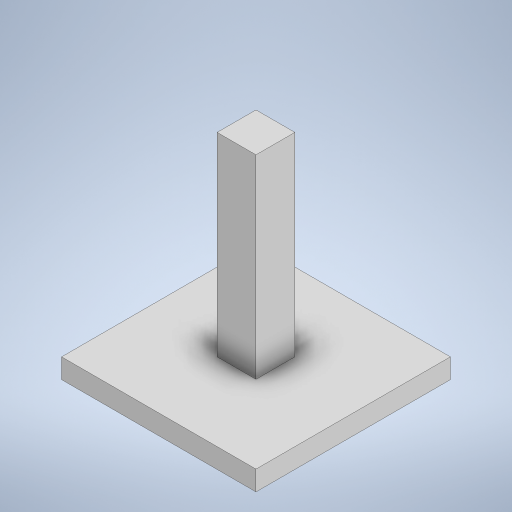
# Autodesk Inventor part: Post
Saved by Autodesk Inventor 2024 (Build 280153000, 153)
## iProperties
Created: 2024-01-14
Part Number: Post
Material: Generic
Document SubType Name: Modeling
Designer: Owner
Density: 1 g/cm^3
Appearance: Default
Author: Owner
Autodesk Inventor part; units mm, degrees
ref_plane "YZ Plane" through (0, 0, 0) normal (1, 0, 0) x (0, 1, 0)
ref_plane "XZ Plane" through (0, 0, 0) normal (0, 1, 0) x (-1, 0, 0)
ref_plane "XY Plane" through (0, 0, 0) normal (0, 0, 1) x (1, 0, 0)
sketch "Sketch1" plane through (0, 0, 0) normal (0, 1, 0) x (-1, 0, 0)
  line L0 (0, 0) -> (500, 0)
  line L1 (500, 0) -> (500, -500)
  line L2 (500, -500) -> (0, -500)
  line L3 (0, -500) -> (0, 0)
  dimension "d0" = 500
  dimension "d1" = 500
  constraints: 8 end point, 2 parallel, 1 horizontal, 1 perpendicular
  measures "d0" distance of L0.end L1.end
  measures "d1" distance of L1.end L2.end
extrude "Extrusion1" add sketch "Sketch1" along normal blind 50.8
sketch "Sketch3" plane through (0, 50.8, 0) normal (0, 1, 0) x (1, 0, 0)
  line L0 (-300, 200) -> (-200, 200)
  line L1 (-200, 200) -> (-200, 300)
  line L2 (-200, 300) -> (-300, 300)
  line L3 (-300, 300) -> (-300, 200)
  line L4 (-300, 200) -> (-200, 300) construction
  line L5 (-200, 200) -> (-300, 300) construction
  line L6 (0, 0) -> (0, 500) projected
  line L7 (-500, 0) -> (0, 0) projected
  point P0 (-250, 250)
  point P1 (-250, 0)
  dimension "d10" = 250
  dimension "d11" = 250
  dimension "d12" = 100
  dimension "d13" = 100
  constraints: 12 end point, 3 midpoint, 2 parallel, 1 horizontal, 1 perpendicular
  measures "d10" distance from line of L6 point (-250, 250)
  measures "d11" distance of point (-250, 0) point (-250, 250)
  measures "d12" distance of L2.end L0.start
  measures "d13" distance of L1.end L2.end
extrude "Extrusion3" add sketch "Sketch3" along normal blind 500
equation "\"d1\" = d0"
equation "\"d11\" = d10"
equation "\"d13\" = d12"
body "Solid1"
